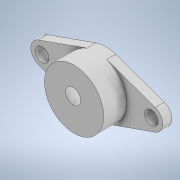
# Autodesk Inventor part: bearingHousing
Saved by Autodesk Inventor 2020 (Build 240168000, 168)
## iProperties
Created: 2022-10-06
Part Number: bearingHousing
Material: Generic
Document SubType Name: Modeling
Designer: karimi2
Density: 1 g/cm^3
Appearance: Default
Author: karimi2
Autodesk Inventor part; units mm, degrees
ref_plane "YZ Plane" through (0, 0, 0) normal (1, 0, 0) x (0, 1, 0)
ref_plane "XZ Plane" through (0, 0, 0) normal (0, 1, 0) x (-1, 0, 0)
ref_plane "XY Plane" through (0, 0, 0) normal (0, 0, 1) x (1, 0, 0)
sketch "Sketch3" plane through (0, 0, 0) normal (0, 0, 1) x (1, 0, 0)
  circle A0 centre (0, 0) radius 5
  circle A1 centre (0, 0) radius 6.5
  line L0 (-12.3755, 0) -> (14, 0) construction
  circle A2 centre (12, 0) radius 2.5
  circle A3 centre (-12, 0) radius 2.5
  line L1 (-12.8333, 2.357) -> (-2.1667, 6.1283)
  line L2 (-12.8333, -2.357) -> (-2.1667, -6.1283)
  line L3 (2.1667, 6.1283) -> (12.8333, 2.357)
  line L4 (12.8333, -2.357) -> (2.1667, -6.1283)
  circle A4 centre (-12, 0) radius 1.5
  circle A5 centre (12, 0) radius 1.5
  dimension "d6" = 10
  dimension "d7" = 13
  dimension "d21" = 5
  dimension "d22" = 5
  dimension "d23" = 12
  dimension "d24" = 12
  dimension "d25" = 3
  dimension "d26" = 3
  constraints: 10 end point, 8 point on circle, 8 tangent, 6 centre point, 4 coincident, 2 point on line, 1 horizontal, 1 parallel
  measures "d6" diameter of A0
  measures "d7" diameter of A1
  measures "d21" diameter of A2
  measures "d22" diameter of A3
  measures "d23" distance of point (0, 0) A3.centre
  measures "d24" distance of A2.centre point (0, 0)
  measures "d25" diameter of A4
  measures "d26" diameter of A5
extrude "Extrusion2" add sketch "Sketch3" along normal blind 7 contours A0 | A1
extrude "Extrusion5" add sketch "Sketch3" along normal blind 2 contours A0 | A1 | A1 L3 A2 L4 | A1 L2 A3 L1 | A2 | A3
sketch "Sketch5" plane through (0, 0, 0) normal (0, 0, -1) x (-1, 0, 0)
  point P0 (0, 0)
  point P1 (0.2154, 0.4635)
hole "Hole2" at (-0.2154, 0.4635, 0) direction (0, 0, 1) diameter 10 depth 5 tip angle 118
body "Solid2"
